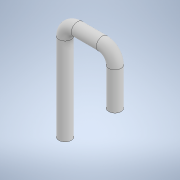
# Autodesk Inventor part: SimpleHook
Saved by Autodesk Inventor 2020.2 (Build 242310000, 310)
## iProperties
Created: 2020-01-08
Part Number: SimpleHook
Material: Generic
Document SubType Name: Modeling
Designer: steele
Density: 1 g/cm^3
Appearance: Default
Author: steele
Autodesk Inventor part; units mm, degrees
ref_plane "YZ Plane" through (0, 0, 0) normal (1, 0, 0) x (0, 1, 0)
ref_plane "XZ Plane" through (0, 0, 0) normal (0, 1, 0) x (-1, 0, 0)
ref_plane "XY Plane" through (0, 0, 0) normal (0, 0, 1) x (1, 0, 0)
sketch "Sketch1" plane through (0, 0, 0) normal (0, 0, 1) x (1, 0, 0)
  line L0 (0, 0) -> (0, 88.9)
  line L1 (12.7, 101.6) -> (38.1, 101.6)
  line L2 (50.8, 88.9) -> (50.8, 50.8)
  arc A0 (12.7, 101.6) -> (0, 88.9) centre (12.7, 88.9) ccw
  arc A1 (50.8, 88.9) -> (38.1, 101.6) centre (38.1, 88.9) ccw
  point P0 (0, 101.6)
  point P1 (50.8, 101.6)
  dimension "d0" = 101.6
  dimension "d1" = 50.8
  dimension "d2" = 50.8
  dimension "d3" = 12.7
  constraints: 6 end point, 4 point on circle, 4 point on line, 4 tangent, 2 centre point, 2 perpendicular, 1 equal radius, 1 vertical
  measures "d0" distance of L0.start point (0, 101.6)
  measures "d1" distance of point (0, 101.6) point (50.8, 101.6)
  measures "d2" distance of point (50.8, 101.6) L2.end
  measures "d3" radius of A0
sketch "Sketch2" plane through (0, 0, 0) normal (0, 1, 0) x (-1, 0, 0)
  circle A0 centre (0, 0) radius 6.35
  dimension "d4" = 12.7
  constraints: 1 centre point, 1 coincident
  measures "d4" diameter of A0
sweep "Sweep1" add profiles "Sketch2" path "Sketch1" path curves L0 A0 L1 A1 L2
body "Solid1"
